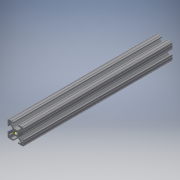
# Autodesk Inventor part: Hook base
Saved by Autodesk Inventor 2018 (Build 220112000, 112)
## iProperties
Company: 80/20 Inc.
Created: 2014-04-23
Part Number: Hook base
Material: Generic
Document SubType Name: Modeling
Density: 1 g/cm^3
Vendor: 80/20 Inc.
Engineer: Ross Bowman
Designer: Ross Bowman
Catalog Web Link: 8020.net
Appearance: Default
Material: 6105-T5 Aluminum
Author: Ross Bowman
Keywords: 80/20 , 8020 , T-Slot , Extrusion
Autodesk Inventor part; units mm, degrees
ref_plane "YZ Plane" through (0, 0, 0) normal (1, 0, 0) x (0, 1, 0)
ref_plane "XZ Plane" through (0, 0, 0) normal (0, 1, 0) x (-1, 0, 0)
ref_plane "XY Plane" through (0, 0, 0) normal (0, 0, 1) x (1, 0, 0)
sketch "Sketch1" plane through (0, 0, 0) normal (0, 0, 1) x (1, 0, 0)
  circle A0 centre (0, 0) radius 2.6035
  arc A1 (-1.7093, -4.4958) -> (-3.9523, -5.4237) centre (-1.7093, -7.6708) ccw
  line L0 (-1.7093, -4.4958) -> (1.7093, -4.4958)
  arc A2 (3.9523, -5.4237) -> (1.7093, -4.4958) centre (1.7093, -7.6708) ccw
  line L1 (3.9523, -5.4237) -> (7.1797, -8.6452)
  arc A3 (6.4164, -10.4902) -> (7.1797, -8.6452) centre (6.4164, -9.4098) ccw
  line L2 (6.4164, -10.4902) -> (4.2875, -10.4902)
  arc A4 (4.2875, -10.4902) -> (3.2385, -11.5392) centre (4.2875, -11.5392) ccw
  line L3 (3.2385, -11.5392) -> (3.2385, -11.651)
  arc A5 (3.2385, -11.651) -> (4.2875, -12.7) centre (4.2875, -11.651) ccw
  line L4 (4.2875, -12.7) -> (5.3171, -12.7)
  arc A6 (6.3331, -12.7) -> (5.3171, -12.7) centre (5.8251, -12.7) ccw
  line L5 (6.3331, -12.7) -> (9.5504, -12.7)
  arc A7 (10.5664, -12.6998) -> (9.5504, -12.7) centre (10.0584, -12.7) ccw
  arc A8 (10.5664, -12.6998) -> (12.6998, -10.5664) centre (10.5918, -10.5918) ccw
  arc A9 (12.7, -9.5504) -> (12.6998, -10.5664) centre (12.7, -10.0584) ccw
  line L6 (12.7, -9.5504) -> (12.7, -6.3331)
  arc A10 (12.7, -5.3171) -> (12.7, -6.3331) centre (12.7, -5.8251) ccw
  line L7 (12.7, -5.3171) -> (12.7, -4.2875)
  arc A11 (12.7, -4.2875) -> (11.651, -3.2385) centre (11.651, -4.2875) ccw
  line L8 (11.651, -3.2385) -> (11.5392, -3.2385)
  arc A12 (11.5392, -3.2385) -> (10.4902, -4.2875) centre (11.5392, -4.2875) ccw
  line L9 (10.4902, -4.2875) -> (10.4902, -6.4021)
  arc A13 (8.7371, -7.1294) -> (10.4902, -6.4021) centre (9.4628, -6.4021) ccw
  line L10 (8.7371, -7.1294) -> (5.441, -3.8408)
  arc A14 (4.5085, -1.5932) -> (5.441, -3.8408) centre (7.6835, -1.5932) ccw
  line L11 (4.5085, -1.5932) -> (4.5085, 1.5932)
  arc A15 (5.441, 3.8408) -> (4.5085, 1.5932) centre (7.6835, 1.5932) ccw
  line L12 (5.441, 3.8408) -> (8.7371, 7.1294)
  arc A16 (10.4902, 6.4021) -> (8.7371, 7.1294) centre (9.4628, 6.4021) ccw
  line L13 (10.4902, 6.4021) -> (10.4902, 4.2875)
  arc A17 (10.4902, 4.2875) -> (11.5392, 3.2385) centre (11.5392, 4.2875) ccw
  line L14 (11.5392, 3.2385) -> (11.651, 3.2385)
  arc A18 (11.651, 3.2385) -> (12.7, 4.2875) centre (11.651, 4.2875) ccw
  line L15 (12.7, 4.2875) -> (12.7, 5.3171)
  arc A19 (12.7, 6.3331) -> (12.7, 5.3171) centre (12.7, 5.8251) ccw
  line L16 (12.7, 6.3331) -> (12.7, 9.5504)
  arc A20 (12.6998, 10.5664) -> (12.7, 9.5504) centre (12.7, 10.0584) ccw
  arc A21 (12.6998, 10.5664) -> (10.5664, 12.6998) centre (10.5918, 10.5918) ccw
  arc A22 (9.5504, 12.7) -> (10.5664, 12.6998) centre (10.0584, 12.7) ccw
  line L17 (9.5504, 12.7) -> (6.3331, 12.7)
  arc A23 (5.3171, 12.7) -> (6.3331, 12.7) centre (5.8251, 12.7) ccw
  line L18 (5.3171, 12.7) -> (4.2875, 12.7)
  arc A24 (4.2875, 12.7) -> (3.2385, 11.651) centre (4.2875, 11.651) ccw
  line L19 (3.2385, 11.651) -> (3.2385, 11.5392)
  arc A25 (3.2385, 11.5392) -> (4.2875, 10.4902) centre (4.2875, 11.5392) ccw
  line L20 (4.2875, 10.4902) -> (6.4768, 10.4902)
  arc A26 (7.207, 8.7244) -> (6.4768, 10.4902) centre (6.4768, 9.4563) ccw
  line L21 (7.207, 8.7244) -> (3.8983, 5.4232)
  arc A27 (1.6558, 4.4958) -> (3.8983, 5.4232) centre (1.6558, 7.6708) ccw
  line L22 (1.6558, 4.4958) -> (-1.6558, 4.4958)
  arc A28 (-3.8983, 5.4232) -> (-1.6558, 4.4958) centre (-1.6558, 7.6708) ccw
  line L23 (-3.8983, 5.4232) -> (-7.207, 8.7244)
  arc A29 (-6.4768, 10.4902) -> (-7.207, 8.7244) centre (-6.4768, 9.4563) ccw
  line L24 (-6.4768, 10.4902) -> (-4.2875, 10.4902)
  arc A30 (-4.2875, 10.4902) -> (-3.2385, 11.5392) centre (-4.2875, 11.5392) ccw
  line L25 (-3.2385, 11.5392) -> (-3.2385, 11.651)
  arc A31 (-3.2385, 11.651) -> (-4.2875, 12.7) centre (-4.2875, 11.651) ccw
  line L26 (-4.2875, 12.7) -> (-5.3171, 12.7)
  arc A32 (-6.3331, 12.7) -> (-5.3171, 12.7) centre (-5.8251, 12.7) ccw
  line L27 (-6.3331, 12.7) -> (-9.5504, 12.7)
  arc A33 (-10.5664, 12.6998) -> (-9.5504, 12.7) centre (-10.0584, 12.7) ccw
  arc A34 (-10.5664, 12.6998) -> (-12.6998, 10.5664) centre (-10.5918, 10.5918) ccw
  arc A35 (-12.7, 9.5504) -> (-12.6998, 10.5664) centre (-12.7, 10.0584) ccw
  line L28 (-12.7, 9.5504) -> (-12.7, 6.3331)
  arc A36 (-12.7, 5.3171) -> (-12.7, 6.3331) centre (-12.7, 5.8251) ccw
  line L29 (-12.7, 5.3171) -> (-12.7, 4.2875)
  arc A37 (-12.7, 4.2875) -> (-11.651, 3.2385) centre (-11.651, 4.2875) ccw
  line L30 (-11.651, 3.2385) -> (-11.5392, 3.2385)
  arc A38 (-11.5392, 3.2385) -> (-10.4902, 4.2875) centre (-11.5392, 4.2875) ccw
  line L31 (-10.4902, 4.2875) -> (-10.4902, 6.4021)
  arc A39 (-8.7371, 7.1294) -> (-10.4902, 6.4021) centre (-9.4628, 6.4021) ccw
  line L32 (-8.7371, 7.1294) -> (-5.441, 3.8408)
  arc A40 (-4.5085, 1.5932) -> (-5.441, 3.8408) centre (-7.6835, 1.5932) ccw
  line L33 (-4.5085, 1.5932) -> (-4.5085, -1.5932)
  arc A41 (-5.441, -3.8408) -> (-4.5085, -1.5932) centre (-7.6835, -1.5932) ccw
  line L34 (-5.441, -3.8408) -> (-8.7371, -7.1294)
  arc A42 (-10.4902, -6.4021) -> (-8.7371, -7.1294) centre (-9.4628, -6.4021) ccw
  line L35 (-10.4902, -6.4021) -> (-10.4902, -4.2875)
  arc A43 (-10.4902, -4.2875) -> (-11.5392, -3.2385) centre (-11.5392, -4.2875) ccw
  line L36 (-11.5392, -3.2385) -> (-11.651, -3.2385)
  arc A44 (-11.651, -3.2385) -> (-12.7, -4.2875) centre (-11.651, -4.2875) ccw
  line L37 (-12.7, -4.2875) -> (-12.7, -5.3171)
  arc A45 (-12.7, -6.3331) -> (-12.7, -5.3171) centre (-12.7, -5.8251) ccw
  line L38 (-12.7, -6.3331) -> (-12.7, -9.5504)
  arc A46 (-12.6998, -10.5664) -> (-12.7, -9.5504) centre (-12.7, -10.0584) ccw
  arc A47 (-12.6998, -10.5664) -> (-10.5664, -12.6998) centre (-10.5918, -10.5918) ccw
  arc A48 (-9.5504, -12.7) -> (-10.5664, -12.6998) centre (-10.0584, -12.7) ccw
  line L39 (-9.5504, -12.7) -> (-6.3331, -12.7)
  arc A49 (-5.3171, -12.7) -> (-6.3331, -12.7) centre (-5.8251, -12.7) ccw
  line L40 (-5.3171, -12.7) -> (-4.2875, -12.7)
  arc A50 (-4.2875, -12.7) -> (-3.2385, -11.651) centre (-4.2875, -11.651) ccw
  line L41 (-3.2385, -11.651) -> (-3.2385, -11.5392)
  arc A51 (-3.2385, -11.5392) -> (-4.2875, -10.4902) centre (-4.2875, -11.5392) ccw
  line L42 (-4.2875, -10.4902) -> (-6.4164, -10.4902)
  arc A52 (-7.1797, -8.6452) -> (-6.4164, -10.4902) centre (-6.4164, -9.4098) ccw
  line L43 (-7.1797, -8.6452) -> (-3.9523, -5.4237)
  constraints: 104 point on circle, 88 end point, 53 centre point
extrude "Extrusion1" add sketch "Sketch1" against normal blind 228.6
sketch "Sketch2" plane through (0, 0, 0) normal (1, 0, 0) x (0, 1, 0)
  point P0 (0, 0)
body "Solid1"
